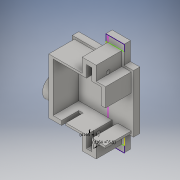
# Autodesk Inventor part: Hip_rotation_temp
Saved by Autodesk Inventor 2016 (Build 200138000, 138)
## iProperties
Created: 2018-07-11
Part Number: Hip_rotation_temp
Material: Generic
Document SubType Name: Modeling
Designer: Attila
Density: 1 g/cm^3
Appearance: Default
Author: Attila
Autodesk Inventor part; units mm, degrees
ref_plane "YZ Plane" through (0, 0, 0) normal (1, 0, 0) x (0, 1, 0)
sketch "Sketch1" plane through (0, 0, 0) normal (0, 0, 1) x (1, 0, 0)
  line L0 (-20, -23) -> (20, -23)
  line L1 (20, -23) -> (20, 23)
  line L2 (20, 23) -> (-20, 23)
  line L3 (-20, 23) -> (-20, -23)
  line L4 (-20, -23) -> (20, 23) construction
  line L5 (20, -23) -> (-20, 23) construction
  point P0 (0, 0)
  dimension "Szelesseg" = 40
  dimension "Magassag" = 46
  constraints: 12 end point, 2 midpoint, 2 parallel, 1 horizontal, 1 perpendicular
  measures "Szelesseg" distance between parallel lines of L1 L3
  measures "Magassag" distance between parallel lines of L0 L2
extrude "Extrusion1" add sketch "Sketch1" along normal blind 3
sketch "Sketch12" plane through (0, 0, 3) normal (0, 0, 1) x (1, 0, 0)
  line L0 (9.3631, -11.3631) -> (5.0131, -11.3631)
  line L1 (5.0131, -11.3631) -> (5.0131, -16.8631)
  line L2 (2.4631, -15.3356) -> (2.4631, -11.3631)
  line L3 (-13.1369, -11.3631) -> (-13.1369, 11.5369)
  line L4 (-13.1369, 11.5369) -> (2.4631, 11.5369)
  line L5 (2.4631, 11.5369) -> (2.4631, 17.0369)
  line L6 (2.4631, 17.0369) -> (5.0131, 17.0369)
  line L7 (5.0131, 17.0369) -> (5.0131, 11.5369)
  line L8 (5.0131, 11.5369) -> (9.3631, 11.5369)
  line L9 (9.3631, 11.5369) -> (9.3631, 3.9369)
  line L10 (7.0131, -12.3631) -> (7.0131, -18.8631)
  line L11 (7.0131, -18.8631) -> (0.4631, -18.8631)
  line L12 (0.4631, -18.8631) -> (0.4631, -12.3631)
  line L13 (-15.1369, -13.3631) -> (-15.1369, 12.5369)
  line L14 (-15.1369, 12.5369) -> (0.4631, 12.5369)
  line L15 (0.4631, 12.5369) -> (0.4631, 19.0369)
  line L16 (0.4631, 19.0369) -> (7.0131, 19.0369)
  line L17 (7.0131, 19.0369) -> (7.0131, 12.5369)
  line L18 (7.0131, 12.5369) -> (11.3631, 12.5369)
  line L19 (11.3631, 12.5369) -> (11.3631, 5.6471)
  line L20 (7.0131, -12.3631) -> (13.6631, -12.3631)
  line L21 (13.6631, -12.3631) -> (13.6631, -11.3631)
  line L22 (13.6631, -11.3631) -> (9.3631, -11.3631)
  line L23 (-9.1369, -13.3631) -> (-9.1369, -11.3631)
  line L24 (-7.1369, -12.3631) -> (-7.1369, -11.3631)
  line L25 (0.4631, -12.3631) -> (-7.1369, -12.3631)
  line L26 (-9.1369, -13.3631) -> (-15.1369, -13.3631)
  line L27 (2.4631, -11.3631) -> (-7.1369, -11.3631)
  line L28 (-9.1369, -11.3631) -> (-13.1369, -11.3631)
  line L29 (-18.3631, -21.3631) -> (-18.3631, 21.3631)
  line L30 (18.3631, 21.3631) -> (18.3631, -21.3631) projected
  line L31 (18.3631, -21.3631) -> (-18.3631, -21.3631) projected
  line L32 (-18.3631, 21.3631) -> (18.3631, 21.3631) projected
  line L33 (2.4631, -15.3356) -> (2.4631, -16.8631)
  line L34 (-16.127, -19.127) -> (16.127, -19.127) projected
  line L35 (2.4631, -16.8631) -> (5.0131, -16.8631)
  line L36 (11.3631, 5.6471) -> (11.3631, 3.9369)
  line L37 (11.3631, 3.9369) -> (9.3631, 3.9369)
  line L38 (-9.1369, -12.3631) -> (-7.1369, -12.3631)
  line L39 (-9.1369, -11.3631) -> (-7.1369, -11.3631)
  point P0 (19.6785, 0.2929)
  dimension "d83" = 22.5
  dimension "d85" = 2.55
  dimension "d86" = 2.55
  dimension "d87" = 15.6
  dimension "d88" = 15.6
  dimension "d89" = 4.35
  dimension "d90" = 4.35
  dimension "d91" = 7.6
  dimension "d92" = 5.5
  dimension "d95" = 22.9
  dimension "d97" = 2
  dimension "d98" = 2
  dimension "d99" = 2
  dimension "d100" = 2
  dimension "d101" = 2
  dimension "d102" = 2
  dimension "d103" = 4.3
  dimension "d105" = 2
  dimension "d106" = 1
  dimension "d107" = 1
  dimension "d109" = 1
  dimension "d110" = 4
  dimension "d111" = 2
  dimension "d112" = 2
  dimension "d113" = 1
  dimension "d114" = 22.9
  dimension "d125" = 2.5
  dimension "d130" = 4.7
  dimension "d132" = 9
  dimension "d133" = 5.5
  dimension "d139" = 2
  constraints: 72 end point, 21 perpendicular, 6 point on line, 3 horizontal, 1 midpoint, 1 vertical
  measures "d83" distance between parallel lines of L9 L3
  measures "d85" distance between parallel lines of L5 L7
  measures "d86" distance between parallel lines of L2 L1
  measures "d87" distance of L3.end L4.end
  measures "d88" distance of L2.end L3.start
  measures "d89" distance of L8.end L7.end
  measures "d90" distance of L0.start L0.end
  measures "d91" distance of L8.end L9.end
  measures "d92" distance between parallel lines of L6 L8
  measures "d95" distance between parallel lines of L8 L0
  measures "d97" distance between parallel lines of L9 L19
  measures "d98" distance between parallel lines of L7 L17
  measures "d99" distance between parallel lines of L16 L6
  measures "d100" distance between parallel lines of L15 L5
  measures "d101" distance between parallel lines of L13 L3
  measures "d102" distance between parallel lines of L10 L1
  measures "d103" distance of L0.start L21.end
  measures "d105" distance between parallel lines of L12 L2
  measures "d106" distance between parallel lines of L18 L8
  measures "d107" distance between parallel lines of L14 L4
  measures "d109" distance between parallel lines of L0 L20
  measures "d110" distance between parallel lines of L3 L23
  measures "d111" distance between parallel lines of L23 L24
  measures "d112" distance between parallel lines of L28 L26
  measures "d113" distance between parallel lines of L27 L25
  measures "d114" distance between parallel lines of L4 L28
  measures "d125" distance between parallel lines of L31 L11
  measures "d130" distance from line of L21.end L30
  measures "d132" distance between parallel lines of L31 L20
  measures "d133" distance between parallel lines of L27 L35
  measures "d139" distance between parallel lines of L35 L11
extrude "Extrusion4" add sketch "Sketch12" along normal blind 12 contours L22 L21 L20 L10 L11 L12 L25 L24 L27 L2 L33 L35 L1 L0 | L24 L38 L23 L39 | L23 L26 L13 L14 L15 L16 L17 L18 L19 L36 L37 L9 L8 L7 L6 L5 L4 L3 L28
sketch "Sketch14" plane through (0, 0, 15) normal (0, 0, 1) x (1, 0, 0)
  line L0 (-9.1369, -12.3631) -> (0.4631, -12.3631) projected
  line L1 (-9.1369, -12.3631) -> (-9.1369, -11.3631)
  line L2 (-13.1369, -11.3631) -> (2.4631, -11.3631) projected
  line L3 (-7.1369, -11.3631) -> (-7.1369, -12.3631)
  point P0 (0, 0)
  dimension "d136" = 2
  constraints: 4 end point, 3 point on line, 1 parallel, 1 vertical
  measures "d136" distance between parallel lines of L3 L1
extrude "Extrusion5" cut sketch "Sketch14" against normal blind 8
sketch "Sketch17" plane through (7.0131, -18.8631, 3) normal (1, 0, 0) x (0, 0, -1)
  line L0 (0, 0) -> (-12, 0) projected
  line L1 (0, 7.5) -> (-12, 7.5) projected
  line L2 (0, 6.5) -> (-12, 6.5) projected
  line L3 (-12, 7.5) -> (-12, 30.4) construction
  line L4 (-12, 18.95) -> (0, 18.95) construction
  line L5 (0, 37.9) -> (-12, 37.9) construction
  line L6 (0, 31.4) -> (-12, 31.4) construction
  point P0 (3, 18.8631)
  point P1 (-6.5, 5.5)
  point P2 (-6.5, 32.4)
  dimension "d144" = 1
  dimension "d145" = 18.95
  dimension "d146" = 1
  constraints: 2 end point, 1 midpoint, 1 perpendicular, 1 symmetric about line
  measures "d144" distance from line of point (-6.5, 5.5) L2
  measures "d145" distance between parallel lines of L5 L4
  measures "d146" distance from line of L6 point (-6.5, 32.4)
hole "Hole3" at (7.0131, -13.3631, 9.5) at (7.0131, 13.5369, 9.5) direction (-1, 0, 0) diameter 1.778 depth 8 tip angle 118
ref_plane "Work Plane1" through (-15.1369, -12.3631, 5) normal (-1, 0, 0) x (0, 0, 1)
sketch "Sketch18" plane through (-15.1369, -12.3631, 5) normal (-1, 0, 0) x (0, 0, 1)
  line L0 (10, 0) -> (0, 0) projected
  line L1 (-2, -9) -> (-2, 33.7262) projected
  circle A0 centre (3.9, 6.9) radius 3.5
  circle A1 centre (3.9, 6.9) radius 5
  point P0 (-5, 12.3631)
  point P1 (9, 0)
  dimension "d156" = 6.9
  dimension "d157" = 5.9
  dimension "d158" = 7
  dimension "d159" = 10
  constraints: 2 centre point, 2 coincident
  measures "d156" distance from line of L0 point (3.9, 6.9)
  measures "d157" distance from line of L1 point (3.9, 6.9)
  measures "d158" diameter of A0
  measures "d159" diameter of A1
extrude "Extrusion6" add sketch "Sketch18" along normal blind 4
sketch "Sketch20" plane through (0, 0, 3) normal (0, 0, 1) x (1, 0, 0)
  point P0 (0, 0)
ref_plane "Work Plane2" through (0.4631, -17.8631, 14) normal (-1, 0, 0) x (0, 0, 1)
sketch "Sketch21" plane through (0.4631, -17.8631, 14) normal (-1, 0, 0) x (0, 0, 1)
  line L0 (-11, -3.5) -> (-11, 39.2262) projected
  arc A0 (-5.389, 4.5) -> (-3.611, 4.5) centre (-4.5, 4.5) ccw projected
  line L1 (0, 5.5) -> (-11, 5.5) projected
  point P0 (-14, 17.8631)
  point P1 (-9, 5.5)
  dimension "d164" = 6.5
  dimension "d165" = 1
  measures "d164" distance from line of L0 A0.centre
  measures "d165" distance from line of L1 A0.centre
sketch "Sketch22" plane through (-15.1369, -13.127, 3) normal (-1, 0, 0) x (0, 0, 1)
  circle A0 centre (5.9, 7.6639) radius 5 projected
  line L0 (5.9, 12.6639) -> (0.0331, 12.6639)
  line L1 (5.9, 2.6639) -> (0.0331, 2.6639)
  line L2 (0.0331, 12.6639) -> (0.0331, 2.6639)
  line L3 (0, -0.2361) -> (0, 25.6639) projected
  point P0 (-3, 13.127)
  point P1 (0, 0)
  point P2 (0, 25.4279)
  point P3 (0, 0.7639)
  point P4 (0, 24.6639)
  constraints: 6 end point, 2 horizontal, 2 point on circle, 2 tangent, 1 parallel
extrude "Extrusion7" add sketch "Sketch22" along normal blind 4 contours A0 L1 L2 L0
sketch "Sketch25" plane through (13.6631, -12.3631, 3) normal (1, 0, 0) x (0, 0, -1)
  line L0 (-12, 1) -> (-12, -4.5) projected
  line L1 (0, 1) -> (-12, 1) projected
  line L2 (-12, -0.0067) -> (0, -0.0067)
  line L3 (0, -0.0067) -> (0, 1)
  line L4 (0, 1) -> (-12, 1)
  line L5 (-12, 1) -> (-12, -0.0067)
  point P0 (3, 12.3631)
  constraints: 8 end point, 2 parallel, 1 horizontal, 1 perpendicular, 1 point on line
extrude "Extrusion8" cut sketch "Sketch25" against normal blind 2.3
sketch "Sketch26" plane through (0, 0, 3) normal (0, 0, 1) x (1, 0, 0)
  line L0 (-19.1369, -13.3631) -> (-19.1369, 2.1817)
  line L1 (-19.1369, -0.4631) -> (-19.1369, -10.4631) projected
  line L2 (-19.1369, 2.1817) -> (-16.1369, 2.1817)
  line L3 (-16.1369, 2.1817) -> (-16.1369, 13.5369)
  line L4 (-16.1369, 13.5369) -> (-0.5369, 13.5369)
  line L5 (-0.5369, 13.5369) -> (-0.5369, 22.0369)
  line L6 (-0.5369, 22.0369) -> (8.0131, 22.0369)
  line L7 (8.0131, 22.0369) -> (8.0131, 13.5369)
  line L8 (8.0131, 13.5369) -> (12.3631, 13.5369)
  line L9 (12.3631, 13.5369) -> (12.3631, -13.3631)
  line L10 (12.3631, -13.3631) -> (8.0131, -13.3631)
  line L11 (8.0131, -13.3631) -> (8.0131, -21.8631)
  line L12 (8.0131, -21.8631) -> (-0.5369, -21.8631)
  line L13 (-0.5369, -21.8631) -> (-0.5369, -13.3631)
  line L14 (-0.5369, -13.3631) -> (-19.1369, -13.3631)
  line L15 (-15.1369, -13.3631) -> (-15.1369, 12.5369) projected
  line L16 (0.4631, 12.5369) -> (-15.1369, 12.5369) projected
  line L17 (0.4631, 19.0369) -> (0.4631, 12.5369) projected
  line L18 (7.0131, 19.0369) -> (0.4631, 19.0369) projected
  line L19 (7.0131, 12.5369) -> (7.0131, 19.0369) projected
  line L20 (11.3631, 3.9369) -> (11.3631, 12.5369) projected
  line L21 (7.0131, -12.3631) -> (11.3631, -12.3631) projected
  line L22 (7.0131, -12.3631) -> (7.0131, -18.8631) projected
  line L23 (0.4631, -18.8631) -> (7.0131, -18.8631) projected
  line L24 (-7.1369, -12.3631) -> (0.4631, -12.3631) projected
  line L25 (-20, -23) -> (20, -23) projected
  line L26 (-20, -23) -> (20, -23)
  line L27 (20, -23) -> (20, 23)
  line L28 (20, 23) -> (-20, 23)
  line L29 (-20, 23) -> (-20, -23)
  point P0 (0, 0)
  dimension "d177" = 1
  dimension "d178" = 1
  dimension "d179" = 1
  dimension "d180" = 3
  dimension "d181" = 1
  dimension "d182" = 1
  dimension "d183" = 1
  dimension "d184" = 1
  dimension "d185" = 3
  dimension "d186" = 1
  dimension "d187" = 4
  dimension "d188" = 3
  constraints: 36 end point, 11 perpendicular, 6 point on line, 2 parallel, 1 collinear, 1 horizontal
  measures "d177" distance between parallel lines of L15 L3
  measures "d178" distance between parallel lines of L4 L16
  measures "d179" distance between parallel lines of L5 L17
  measures "d180" distance between parallel lines of L6 L18
  measures "d181" distance between parallel lines of L19 L7
  measures "d182" distance between parallel lines of L9 L20
  measures "d183" distance between parallel lines of L10 L21
  measures "d184" distance between parallel lines of L22 L11
  measures "d185" distance between parallel lines of L23 L12
  measures "d186" distance between parallel lines of L14 L24
  measures "d187" distance between parallel lines of L0 L15
  measures "d188" distance of L0.end L2.end
extrude "Extrusion9" cut sketch "Sketch26" against normal blind 10
sketch "Sketch27" plane through (0, 0, 3) normal (0, 0, 1) x (1, 0, 0)
  line L0 (-0.5369, 22.0369) -> (-0.5369, 13.5369) projected
  line L1 (8.0131, 22.0369) -> (-0.5369, 22.0369) projected
  line L2 (-0.5369, 19.0369) -> (8.0131, 19.0369)
  line L3 (8.0131, 19.0369) -> (8.0131, 22.0369)
  line L4 (8.0131, 22.0369) -> (-0.5369, 22.0369)
  line L5 (-0.5369, 22.0369) -> (-0.5369, 19.0369)
  line L6 (-0.5369, -21.8631) -> (-0.5369, -13.3631) projected
  line L7 (8.0131, -21.8631) -> (8.0131, -13.3631) projected
  line L8 (-0.5369, -21.8631) -> (8.0131, -21.8631)
  line L9 (8.0131, -21.8631) -> (8.0131, -18.8631)
  line L10 (8.0131, -18.8631) -> (-0.5369, -18.8631)
  line L11 (-0.5369, -18.8631) -> (-0.5369, -21.8631)
  point P0 (0, 0)
  constraints: 16 end point, 4 parallel, 2 horizontal, 2 perpendicular, 2 point on line
equation "\"d86\" = d85"
equation "\"d90\" = d89"
equation "\"d95\" = d82"
equation "\"d9\" = 0.5 * d10"
equation "\"d12\" = d11"
equation "\"d13\" = d11"
equation "\"d14\" = d11"
equation "\"d93\" = d92"
equation "\"d82\" = 22.9"
equation "\"d10\" = 18.133333"
equation "\"d11\" = 2"
body "Solid1"
